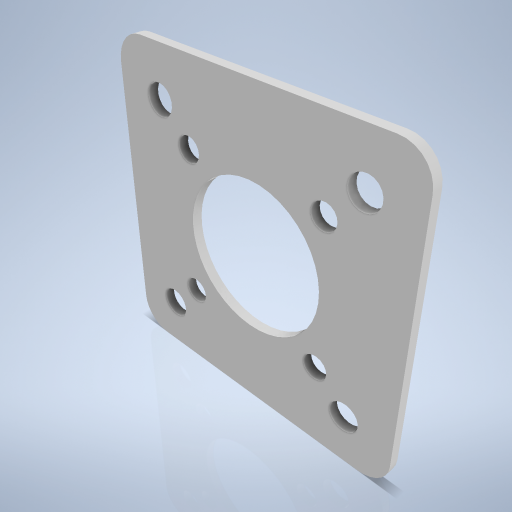
# Autodesk Inventor part: 12
Saved by Autodesk Inventor 2024.2 (Build 282272000, 272)
## iProperties
Created: 2024-05-14
Part Number: 12
Material: Generisch
Document SubType Name: Modeling
Designer: Fabri
Density: 1 g/cm^3
Appearance: Vorgabe
Author: Fabri
Autodesk Inventor part; units mm, degrees
ref_plane "YZ Plane" through (0, 0, 0) normal (1, 0, 0) x (0, 1, 0)
ref_plane "XZ Plane" through (0, 0, 0) normal (0, 1, 0) x (-1, 0, 0)
ref_plane "XY Plane" through (0, 0, 0) normal (0, 0, 1) x (1, 0, 0)
sketch "Skizze1" plane through (0, 0, 0) normal (0, 1, 0) x (-1, 0, 0)
  line L0 (31, 31) -> (-31, 31)
  line L1 (-31, 31) -> (-31, -31)
  line L2 (-31, -31) -> (31, -31)
  line L3 (31, -31) -> (31, 31)
  line L4 (31, 31) -> (-31, -31) construction
  line L5 (-31, 31) -> (31, -31) construction
  point P0 (0, 0)
  dimension "d0" = 62
  dimension "d1" = 62
  constraints: 12 end point, 2 midpoint, 2 parallel, 1 horizontal, 1 perpendicular
  measures "d0" distance of L2.end L1.end
  measures "d1" distance of L1.end L0.end
extrude "Extrusion1" add sketch "Skizze1" along normal blind 2
fillet "Rundung1" radius 6 4 edges at (-31, 1, 31) (31, 1, 31) (31, 1, -31) (-31, 1, -31)
sketch "Skizze2" plane through (0, 2, 0) normal (0, 1, 0) x (1, 0, 0)
  line L0 (-25, -31) -> (25, -31) projected
  line L1 (0, -31) -> (0, 31) construction
  line L2 (25, 31) -> (-25, 31) projected
  line L3 (31, -25) -> (31, 25) projected
  line L4 (31, 0) -> (-31, 0) construction
  line L5 (-31, 25) -> (-31, -25) projected
  point P0 (0, 0)
  point P1 (21.124, 21.124)
  point P2 (21.124, -21.124)
  point P3 (-21.124, 21.124)
  point P4 (-21.124, -21.124)
  dimension "d37" = 42.248
  dimension "d38" = 42.248
  dimension "d39" = 42.248
  constraints: 4 end point, 4 midpoint, 2 horizontal alignment, 2 symmetric about line, 1 vertical alignment
  measures "d37" distance of point (-21.124, 21.124) point (21.124, 21.124)
  measures "d38" distance of point (21.124, 21.124) point (21.124, -21.124)
  measures "d39" distance of point (-21.124, -21.124) point (21.124, -21.124)
hole "Bohrung1" at (21.124, 2, -21.124) at (21.124, 2, 21.124) at (-21.124, 2, -21.124) at (-21.124, 2, 21.124) direction (0, -1, 0) diameter 6 depth 2
hole "Bohrung2" at (0, 2, 0) direction (0, -1, 0) diameter 29 depth 2
sketch "Skizze3" plane through (0, 0, 0) normal (0, -1, 0) x (1, 0, 0)
  point P0 (0, 0)
  point P1 (-14.5, 14.5)
  point P2 (14.5, 14.5)
  point P3 (-14.5, -14.5)
  point P4 (14.5, -14.5)
  dimension "d33" = 29
  dimension "d34" = 14.5
  dimension "d35" = 29
  dimension "d36" = 14.5
  constraints: 2 horizontal alignment, 2 vertical alignment
  measures "d33" distance of point (-14.5, -14.5) point (-14.5, 14.5)
  measures "d34" horizontal distance of point (0, 0) point (-14.5, 14.5)
  measures "d35" distance of point (14.5, 14.5) point (-14.5, 14.5)
  measures "d36" horizontal distance of point (0, 0) point (14.5, 14.5)
hole "Bohrung3" at (-14.5, 0, 14.5) at (14.5, 0, 14.5) at (-14.5, 0, -14.5) at (14.5, 0, -14.5) direction (0, 1, 0) diameter 5 depth 2
equation "\"d37\" = d38"
equation "\"d39\" = d38"
